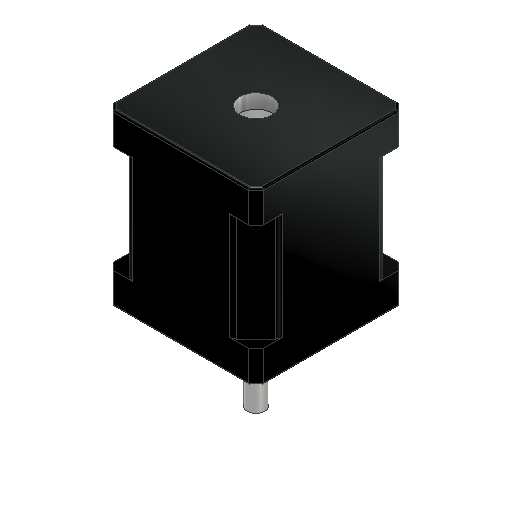
# Autodesk Inventor part: COTS_GENERIC_NEMA17_25mm_shaft
Saved by Autodesk Inventor 2026.1 (Build 301233000, 233)
## iProperties
Created: 2016-01-19
Part Number: COTS_GENERIC_NEMA17_25mm_shaft
Material: Ogólny
Document SubType Name: Modeling
Designer: Andrzej
Density: 1 g/cm^3
Appearance: Brąz armatni - polerowany
Mass: 82.4142 g
Surface Area: 120.186 cm^2
Volume: 82.4142 cm^3
Author: Andrzej
Autodesk Inventor part; units mm, degrees
ref_plane "YZ Plane" through (0, 0, 0) normal (1, 0, 0) x (0, 1, 0)
ref_plane "XZ Plane" through (0, 0, 0) normal (0, 1, 0) x (-1, 0, 0)
ref_plane "XY Plane" through (0, 0, 0) normal (0, 0, 1) x (1, 0, 0)
sketch "Szkic1" plane through (0, 0, 0) normal (0, 0, 1) x (1, 0, 0)
  line L0 (-18.7306, 19.0987) -> (23.2694, 19.0987)
  line L1 (23.2694, 19.0987) -> (23.2694, -22.9013)
  line L2 (23.2694, -22.9013) -> (-18.7306, -22.9013)
  line L3 (-18.7306, -22.9013) -> (-18.7306, 19.0987)
  point P0 (0, 0)
  dimension "d0" = 42
  dimension "d1" = 42
  constraints: 8 end point, 2 parallel, 1 horizontal, 1 perpendicular
  measures "d0" distance of L1.end L2.end
  measures "d1" distance of L0.end L1.end
extrude "Wyciągnięcie proste1" add sketch "Szkic1" along normal blind 9
chamfer "Faza1" distance 2 angle 45 4 edges at (23.2694, 19.0987, 4.5) (-18.7306, 19.0987, 4.5) (-18.7306, -22.9013, 4.5) (23.2694, -22.9013, 4.5)
sketch "Szkic2" plane through (0, 0, 0) normal (0, 0, -1) x (-1, 0, 0)
  line L0 (-21.2694, -22.9013) -> (-23.2694, -20.9013) projected
  line L1 (-21.2694, -22.9013) -> (16.7306, -22.9013) projected
  line L2 (18.7306, -20.9013) -> (16.7306, -22.9013) projected
  line L3 (18.7306, -20.9013) -> (18.7306, 17.0987) projected
  line L4 (16.7306, 19.0987) -> (18.7306, 17.0987) projected
  line L5 (16.7306, 19.0987) -> (-21.2694, 19.0987) projected
  line L6 (-23.2694, 17.0987) -> (-21.2694, 19.0987) projected
  line L7 (-23.2694, 17.0987) -> (-23.2694, -20.9013) projected
  line L8 (12.0859, 19.0987) -> (-16.6247, 19.0987)
  line L9 (-23.2694, -16.2567) -> (-16.6247, -22.9013)
  line L10 (12.0859, -22.9013) -> (18.7306, -16.2567)
  line L11 (-23.2694, 12.454) -> (-16.6247, 19.0987)
  line L12 (12.0859, 19.0987) -> (18.7306, 12.454)
  line L13 (-16.6247, 19.0987) -> (12.0859, 19.0987)
  line L14 (-23.2694, 17.0987) -> (-23.2694, -20.9013) projected
  line L15 (-23.2694, 12.454) -> (-23.2694, -16.2567)
  line L16 (-23.2694, -16.2567) -> (-23.2694, 12.454)
  line L17 (-16.6247, -22.9013) -> (12.0859, -22.9013)
  line L18 (-16.6247, -22.9013) -> (12.0859, -22.9013)
  line L19 (18.7306, -16.2567) -> (18.7306, 12.454)
  point P0 (0, 0)
  point P1 (-2.2694, -1.9013)
  dimension "d9" = 21
  dimension "d10" = 42
  dimension "d11" = 21
  dimension "d12" = 25
  dimension "d13" = 25
  dimension "d14" = 25
  dimension "d15" = 25
  constraints: 25 end point, 3 collinear, 2 perpendicular, 1 parallel, 1 point on line
  measures "d9" distance from line of point (-2.269, -1.901) L7
  measures "d10" distance between parallel lines of L3 L7
  measures "d11" distance from line of L5 point (-2.269, -1.901)
  measures "d12" distance from line of L9 point (-2.269, -1.901)
  measures "d13" distance from line of L12 point (-2.269, -1.901)
  measures "d14" distance from line of L11 point (-2.269, -1.901)
  measures "d15" distance from line of L10 point (-2.269, -1.901)
extrude "Wyciągnięcie proste3" add sketch "Szkic2" along normal blind 30 contours L9 L7 L11 L5 L12 L3 L10 L1
sketch "Szkic3" plane through (0, 0, -30) normal (0, 0, -1) x (-1, 0, 0)
  line L0 (-23.2694, -16.2567) -> (-16.6247, -22.9013) projected
  line L1 (-16.6247, -22.9013) -> (12.0859, -22.9013) projected
  line L2 (12.0859, -22.9013) -> (18.7306, -16.2567) projected
  line L3 (18.7306, -16.2567) -> (18.7306, 12.454) projected
  line L4 (18.7306, 12.454) -> (12.0859, 19.0987) projected
  line L5 (12.0859, 19.0987) -> (-16.6247, 19.0987) projected
  line L6 (-16.6247, 19.0987) -> (-23.2694, 12.454) projected
  line L7 (-23.2694, 12.454) -> (-23.2694, -16.2567) projected
  line L8 (-23.2694, 12.454) -> (-16.6247, 19.0987) projected
  line L9 (-16.6247, 19.0987) -> (-21.2694, 19.0987) projected
  line L10 (-23.2694, 17.0987) -> (-21.2694, 19.0987) projected
  line L11 (-23.2694, 17.0987) -> (-23.2694, 12.454) projected
  line L12 (-16.6247, -22.9013) -> (-23.2694, -16.2567) projected
  line L13 (-23.2694, -16.2567) -> (-23.2694, -20.9013) projected
  line L14 (-21.2694, -22.9013) -> (-23.2694, -20.9013) projected
  line L15 (-21.2694, -22.9013) -> (-16.6247, -22.9013) projected
  line L16 (18.7306, -16.2567) -> (12.0859, -22.9013) projected
  line L17 (12.0859, -22.9013) -> (16.7306, -22.9013) projected
  line L18 (18.7306, -20.9013) -> (16.7306, -22.9013) projected
  line L19 (18.7306, -20.9013) -> (18.7306, -16.2567) projected
  line L20 (12.0859, 19.0987) -> (18.7306, 12.454) projected
  line L21 (18.7306, 12.454) -> (18.7306, 17.0987) projected
  line L22 (16.7306, 19.0987) -> (18.7306, 17.0987) projected
  line L23 (16.7306, 19.0987) -> (12.0859, 19.0987) projected
  line L24 (-23.2694, 19.0987) -> (-23.2694, -22.9013)
  line L25 (-23.2694, -22.9013) -> (18.7306, -22.9013)
  line L26 (18.7306, -22.9013) -> (18.7306, 19.0987)
  line L27 (18.7306, 19.0987) -> (-23.2694, 19.0987)
  point P0 (0, 0)
  constraints: 8 end point, 1 perpendicular, 1 point on line
extrude "Wyciągnięcie proste4" add sketch "Szkic3" along normal blind 9 contours L7 L6 L5 L4 L3 L2 L1 L0 | L0 L15 L14 L13 | L11 L10 L9 L6 | L2 L19 L18 L17 | L23 L22 L21 L4
fillet "Zaokrąglenie1" radius 2 8 edges at (-18.7306, 12.454, -15) (-12.0859, 19.0987, -15) (16.6247, 19.0987, -15) (23.2694, 12.454, -15) (-18.7306, -16.2567, -15) (-12.0859, -22.9013, -15) (16.6247, -22.9013, -15) (23.2694, -16.2567, -15)
sketch "Szkic4" plane through (0, 0, 9) normal (0, 0, 1) x (1, 0, 0)
  line L0 (-18.7306, 17.0987) -> (-18.7306, -20.9013) projected
  line L1 (23.2694, -20.9013) -> (23.2694, 17.0987) projected
  line L2 (21.2694, 19.0987) -> (-16.7306, 19.0987) projected
  circle A0 centre (2.2694, -1.9013) radius 4.5
  line L3 (23.2694, 19.0987) -> (-18.7306, 19.0987)
  line L4 (23.2694, -22.9013) -> (-18.7306, -22.9013)
  line L5 (21.2694, -22.9013) -> (-16.7306, -22.9013) projected
  line L6 (-18.7306, -22.9013) -> (-18.7306, 19.0987)
  line L7 (23.2694, 19.0987) -> (23.2694, -22.9013)
  point P0 (0, 0)
  dimension "d21" = 42
  dimension "d22" = 21
  dimension "d23" = 21
  dimension "d24" = 9
  constraints: 8 end point, 3 collinear, 1 centre point, 1 coincident, 1 point on line
  measures "d21" distance between parallel lines of L0 L1
  measures "d22" distance from line of L2 point (2.269, -1.901)
  measures "d23" distance from line of L1 point (2.269, -1.901)
  measures "d24" diameter of A0
extrude "Wyciągnięcie proste5" cut sketch "Szkic4" against normal blind 4 contours A0
fillet "Zaokrąglenie2" radius 0.6 16 edges at (23.2694, -1.9013, 9) (2.2694, -22.9013, 9) (-18.7306, -1.9013, 9) (2.2694, 19.0987, 9) (22.2694, -21.9013, 9) (-17.7306, -21.9013, 9) (-17.7306, 18.0987, 9) (22.2694, 18.0987, 9) (23.2694, -1.9013, -39) (22.2694, 18.0987, -39) (2.2694, 19.0987, -39) (-17.7306, 18.0987, -39) (-18.7306, -1.9013, -39) (-17.7306, -21.9013, -39) (2.2694, -22.9013, -39) (22.2694, -21.9013, -39)
sketch "Szkic5" plane through (0, 0, -39) normal (0, 0, -1) x (-1, 0, 0)
  circle A0 centre (-2.2694, -1.9013) radius 4.5 projected
  line L0 (-21.2694, -22.9013) -> (16.7306, -22.9013) projected
  line L1 (16.7306, -22.9013) -> (18.7306, -20.9013) projected
  line L2 (18.7306, -20.9013) -> (18.7306, 17.0987) projected
  line L3 (18.7306, 17.0987) -> (16.7306, 19.0987) projected
  line L4 (16.7306, 19.0987) -> (-21.2694, 19.0987) projected
  line L5 (-21.2694, 19.0987) -> (-23.2694, 17.0987) projected
  line L6 (-23.2694, 17.0987) -> (-23.2694, -20.9013) projected
  line L7 (-23.2694, -20.9013) -> (-21.2694, -22.9013) projected
  line L8 (18.7306, -22.9013) -> (18.7306, 19.0987)
  line L9 (18.7306, 19.0987) -> (-23.2694, 19.0987)
  line L10 (-23.2694, 19.0987) -> (-23.2694, -22.9013)
  line L11 (-23.2694, -22.9013) -> (18.7306, -22.9013)
  circle A1 centre (-2.2694, -1.9013) radius 11
  circle A2 centre (-2.2694, -1.9013) radius 16.25
  circle A3 centre (-2.2694, -1.9013) radius 2.5
  point P0 (0, 0)
  point P1 (13.1806, -17.3513)
  point P2 (13.1806, 13.5487)
  point P3 (-17.7194, 13.5487)
  point P4 (-17.7194, -17.3513)
  dimension "d28" = 42
  dimension "d29" = 5.55
  dimension "d30" = 5.55
  dimension "d31" = 5.55
  dimension "d32" = 5.55
  dimension "d33" = 5.55
  dimension "d34" = 5.55
  dimension "d35" = 5.55
  dimension "d36" = 5.55
  dimension "d37" = 22
  dimension "d38" = 32.5
  dimension "d53" = 5
  constraints: 8 end point, 3 centre point, 1 coincident, 1 collinear, 1 perpendicular, 1 point on line, 1 vertical
  measures "d28" distance between parallel lines of L4 L0
  measures "d29" distance from line of L0 point (13.181, -17.351)
  measures "d30" distance from line of L4 point (13.181, 13.549)
  measures "d31" distance from line of L2 point (13.181, 13.549)
  measures "d32" distance from line of L4 point (-17.719, 13.549)
  measures "d33" distance from line of L6 point (-17.719, 13.549)
  measures "d34" distance from line of L6 point (-17.719, -17.351)
  measures "d35" distance from line of L0 point (-17.719, -17.351)
  measures "d36" distance from line of L2 point (13.181, -17.351)
  measures "d37" diameter of A1
  measures "d38" diameter of A2
  measures "d53" diameter of A3
extrude "Wyciągnięcie proste6" cut sketch "Szkic5" against normal blind 0.3 contours A2
extrude "Wyciągnięcie proste7" add sketch "Szkic5" along normal blind 2 contours A1
chamfer "Faza2" distance 0.5 angle 45 1 edges at (6.7694, -1.9013, -41)
hole "Otwór1" at (-13.1806, -17.3513, -39) at (-13.1806, 13.5487, -39) at (17.7194, 13.5487, -39) at (17.7194, -17.3513, -39) direction (0, 0, 1) diameter 3 depth 5 tip angle 118
extrude "Wyciągnięcie proste8" add sketch "Szkic5" along normal blind 25 contours A3
equation "\"d13\" = d12"
equation "\"d14\" = d12"
equation "\"d15\" = d12"
equation "\"d22\" = 0.5 * d21"
equation "\"d23\" = 0.5 * d21"
equation "\"d30\" = d29"
equation "\"d31\" = d29"
equation "\"d32\" = d29"
equation "\"d33\" = d31"
equation "\"d34\" = d29"
equation "\"d35\" = d29"
equation "\"d36\" = d29"
